Autodesk Fusion 360 part; units mm, degrees
(part 2 of 2)
sketch "Sketch1 (3)" plane through (0, -4, 0) normal (0, 1, 0) x (-1, 0, 0) in component "Window"
  line L0 (-24.907, 84.996) -> (-24.907, 43.878)
  arc A0 (-24.907, 43.878) -> (-13.907, 32.878) centre (-13.907, 43.878) ccw
  line L1 (-13.907, 32.878) -> (-9.873, 32.878)
  arc A1 (-6.873, 29.878) -> (-9.873, 32.878) centre (-9.873, 29.878) ccw
  line L2 (-6.873, 29.878) -> (-6.873, 10)
  arc A2 (-9.873, 7) -> (-6.873, 10) centre (-9.873, 10) ccw
  line L3 (-9.873, 7) -> (-84.361, 7)
  arc A3 (-87.361, 10) -> (-84.361, 7) centre (-84.361, 10) ccw
  line L4 (-87.361, 10) -> (-87.361, 84.996)
  arc A4 (-84.361, 87.996) -> (-87.361, 84.996) centre (-84.361, 84.996) ccw
  line L5 (-84.361, 87.996) -> (-27.907, 87.996)
  arc A5 (-24.907, 84.996) -> (-27.907, 87.996) centre (-27.907, 84.996) ccw
  line L6 (-19.407, 43.878) -> (-19.407, 91.5154)
  arc A6 (-19.407, 91.5154) -> (-21.685, 93.496) centre (-19.685, 93.496) ccw
  line L7 (-21.685, 93.496) -> (-90.837, 93.496)
  arc A7 (-90.837, 93.496) -> (-92.861, 91.4961) centre (-92.837, 93.496) ccw
  line L8 (-92.861, 91.4961) -> (-92.861, 3.778)
  arc A8 (-92.861, 3.778) -> (-90.8804, 1.5) centre (-92.861, 1.778) ccw
  line L9 (-90.8804, 1.5) -> (-3.397, 1.5)
  arc A9 (-3.397, 1.5) -> (-1.373, 3.4999) centre (-1.397, 1.5) ccw
  line L10 (-1.373, 3.4999) -> (-1.373, 36.378)
  arc A10 (-1.373, 36.378) -> (-3.373, 38.378) centre (-1.373, 38.378) ccw
  line L11 (-3.373, 38.378) -> (-13.907, 38.378)
  arc A11 (-19.407, 43.878) -> (-13.907, 38.378) centre (-13.907, 43.878) ccw
  line L12 (1.127, 38.608) -> (1.127, 1.524) construction
  arc A12 (1.127, 38.608) -> (-1.143, 40.878) centre (-1.143, 38.608) ccw construction
  line L13 (-13.907, 40.878) -> (-1.143, 40.878) construction
  arc A13 (-16.907, 43.878) -> (-13.907, 40.878) centre (-13.907, 43.878) ccw construction
  line L14 (-16.907, 93.218) -> (-16.907, 43.878) construction
  arc A14 (-16.907, 93.218) -> (-19.685, 95.996) centre (-19.685, 93.218) ccw construction
  line L15 (-92.837, 95.996) -> (-19.685, 95.996) construction
  arc A15 (-92.837, 95.996) -> (-95.361, 93.472) centre (-92.837, 93.472) ccw construction
  line L16 (-95.361, 1.778) -> (-95.361, 93.472) construction
  arc A16 (-95.361, 1.778) -> (-92.583, -1) centre (-92.583, 1.778) ccw construction
  line L17 (-1.397, -1) -> (-92.583, -1) construction
  arc A17 (-1.397, -1) -> (1.127, 1.524) centre (-1.397, 1.524) ccw construction
  line L18 (-2.048, 37.703) -> (-2.048, 2.175)
  line L19 (-13.907, 37.703) -> (-2.048, 37.703)
  arc A18 (-20.082, 43.878) -> (-13.907, 37.703) centre (-13.907, 43.878) ccw
  line L20 (-20.082, 92.821) -> (-20.082, 43.878)
  line L21 (-92.186, 92.821) -> (-20.082, 92.821)
  line L22 (-92.186, 2.175) -> (-92.186, 92.821)
  line L23 (-2.048, 2.175) -> (-92.186, 2.175)
  dimension "d49" = -3.175
extrude "Extrude1'''" add sketch "Sketch1 (3)" along normal blind 3 separate body contours L0 A0 L1 A1 L2 A2 L3 A3 L4 A4 L5 A5 | L18 L19 A18 L20 L21 L22 L23 makes body 4 in component "Window"
component "MidLayer" placed x (1, 0, 0) y (0, 1, 0) z (0, 0, 1) at (0, 0, 0)
component "TopLayer" placed x (1, 0, 0) y (0, 1, 0) z (0, 0, 1) at (0, 0, 0)
component "BaseLayer" placed x (1, 0, 0) y (0, 1, 0) z (0, 0, 1) at (0, 0, 0)
component "Window" placed x (1, 0, 0) y (0, 1, 0) z (0, 0, 1) at (0, 0, 0)
equation "mx_dim = 14.05 mm" comment "Cherry MX holes dimensions"
equation "t_spacing = 0.5 mm" comment "Tight spacing"
equation "n_spacing = 1 mm" comment "Normal spacing"
equation "m4_dim = 4.3 mm" comment "M4 screws dimensions"
equation "acrylic_h = 3 mm" comment "Acrylic sheet height"
equation "mdf_h = 6 mm" comment "MDF sheet height"
equation "d7 = n_spacing"
equation "d8 = n_spacing + border_dim"
equation "border_dim = 5 mm" comment "Border dimensions"
equation "d12 = acrylic_h"
equation "d14 = mx_dim"
equation "d15 = mx_dim"
equation "d16 = mx_dim"
equation "d17 = mx_dim"
equation "d18 = mx_dim"
equation "d19 = mx_dim"
equation "d20 = mx_dim"
equation "d21 = mx_dim"
equation "d24 = mdf_h"
equation "d26 = t_spacing"
equation "d30 = -mdf_h"
equation "d35 = -3 mm - 5 mm"
equation "d50 = acrylic_h"
